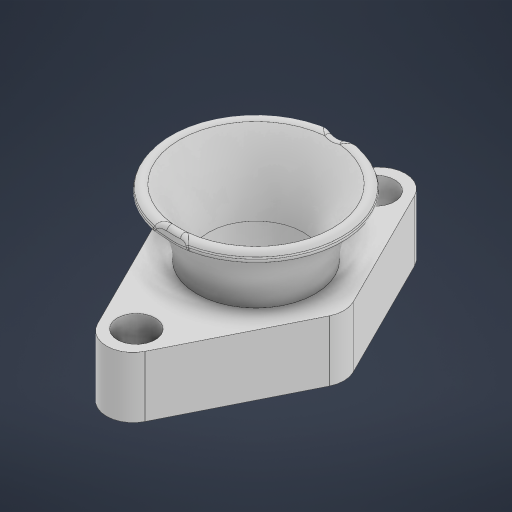
# Autodesk Inventor part: velocity stack
Saved by Autodesk Inventor 2024.2 (Build 282272000, 272)
## iProperties
Created: 2025-06-20
Part Number: velocity stack
Material: Generic
Document SubType Name: Modeling
Designer: Moe
Density: 1 g/cm^3
Appearance: Default
Author: Moe
Autodesk Inventor part; units mm, degrees
ref_plane "YZ Plane" through (0, 0, 0) normal (1, 0, 0) x (0, 1, 0)
ref_plane "XZ Plane" through (0, 0, 0) normal (0, 1, 0) x (-1, 0, 0)
sketch "Sketch1" plane through (0, 0, 0) normal (0, 1, 0) x (-1, 0, 0)
  circle A0 centre (0, 0) radius 6.25
  circle A1 centre (0, -15.75) radius 2.5
  circle A2 centre (0, 15.75) radius 2.5
  line L0 (0, 0) -> (0, -24)
  line L1 (0, 0) -> (0, 24)
  line L2 (0, 0) -> (12, 0)
  line L3 (0, 0) -> (-12, 0)
  line L4 (0, 24) -> (12, 0)
  line L5 (12, 0) -> (0, -24)
  line L6 (0, -24) -> (-12, 0)
  line L7 (-12, 0) -> (0, 24)
  line L8 (12.016091, 26.451229) -> (-11.988013, 26.451229)
  line L9 (-11.988013, 26.451229) -> (-11.988013, 27.744681)
  line L10 (-11.988013, 27.744681) -> (12.016091, 27.744681)
  line L11 (12.016091, 27.744681) -> (12.016091, 26.451229)
  dimension "d0" = 12.5
  dimension "d1" = 5
  dimension "d2" = 5
  dimension "d3" = 15.75
  dimension "d4" = 15.75
  dimension "d5" = 24
  dimension "d6" = 24
  dimension "d7" = 12
  dimension "d8" = 12
  constraints: 24 end point, 3 centre point, 3 horizontal, 2 parallel, 2 vertical, 1 coincident, 1 perpendicular
  measures "d0" diameter of A0
  measures "d1" diameter of A1
  measures "d2" diameter of A2
  measures "d3" distance of point (0, 0) A2.centre
  measures "d4" distance of A1.centre point (0, 0)
  measures "d5" distance of L0.start L0.end
  measures "d6" distance of L0.start L1.end
  measures "d7" distance of L0.start L2.end
  measures "d8" distance of L0.start L3.end
extrude "Extrusion1" add sketch "Sketch1" along normal blind 8 contours L2 L5 L0 A1 A0 | A0 L1 A2 L4 L2 | A0 L3 L7 L1 A2 | L0 A1 L6 L3 A0
fillet "Fillet1" radius 3.5 4 edges at (0, 4, 24) (0, 4, -24) (12, 4, 0) (-12, 4, 0)
sketch "Sketch2" plane through (0, 0, 0) normal (0, -1, 0) x (1, 0, 0)
  circle A0 centre (0, 0) radius 6.25 projected
  circle A1 centre (0, 0) radius 10
  dimension "d12" = 20
  constraints: 1 centre point, 1 coincident
  measures "d12" diameter of A1
extrude "Extrusion2" cut sketch "Sketch2" against normal blind 3.5
extrude "Extrusion3" add sketch "Sketch1" along normal blind 10 contours L8 L9 L10 L11
ref_plane "Work Plane2" through (11.988013, 0, 0.000229) normal (0, 0, -1) x (-1, 0, 0)
extrude "Extrusion4" cut sketch "Sketch1" along normal blind 10 contours L8 L9 L10 L11
sketch "Sketch4" plane through (11.988013, 0, 0.000229) normal (0, 0, -1) x (-1, 0, 0)
  line L0 (23.205389, 8) -> (23.205389, 8)
  line L1 (23.205389, 8) -> (15.118508, 8)
  line L2 (8.857518, 8) -> (15.118508, 8)
  line L3 (8.857518, 8) -> (0.770637, 8)
  line L4 (0.770637, 8) -> (0.770637, 8)
  line L5 (0.770637, 8) -> (8.857518, 8)
  line L6 (15.118508, 8) -> (8.857518, 8)
  line L7 (15.118508, 8) -> (23.205389, 8)
  line L8 (9.488013, 8) -> (14.488013, 8)
  line L9 (9.488013, 8) -> (14.488013, 8)
  line L10 (5.738013, 8) -> (18.238013, 8)
  line L11 (5.738013, 3.5) -> (18.238013, 3.5)
  line L12 (5.738013, 8) -> (18.238013, 8)
  arc A0 (22.062221, 16.642429) -> (18.238013, 8) centre (29.105693, 8.358441) ccw
  line L13 (18.238013, 8) -> (23.982272, 17.949349) construction
  line L14 (18.238013, 8) -> (29.726531, 8) construction
  line L15 (23.205389, 8) -> (15.118508, 8)
  line L16 (19.793316, 8) -> (18.238013, 8)
  line L17 (11.988013, 0) -> (11.988013, 10.466692)
  arc A1 (23.281166, 15.663138) -> (19.779795, 7.800469) centre (29.105693, 8.358441) ccw
  line L18 (23.326048, 16.322868) -> (23.4046, 16.120844)
  arc A2 (23.326048, 16.322868) -> (22.062221, 16.642429) centre (22.580428, 16.032953) ccw
  arc A3 (23.281166, 15.663138) -> (23.4046, 16.120844) centre (23.03179, 15.975886) ccw
  point P0 (22.940237, 17.31512)
  point P1 (23.512979, 15.842108)
  point P2 (19.769997, 8)
  dimension "d22" = 60
  dimension "d26" = 0.8
  dimension "d27" = 0.4
  constraints: 11 point on circle, 10 end point, 4 centre point, 4 tangent, 3 point on line, 1 coincident, 1 collinear, 1 equal length, 1 horizontal, 1 vertical
  measures "d22" angle of L14 L13
  measures "d26" radius of A2
  measures "d27" radius of A3
revolve "Revolution1" add sketch "Sketch4" angle 360 about axis through (0, 0, 0.000229) along (0, 1, 0)
sketch "Sketch5" plane through (0, 8, 0) normal (0, 1, 0) x (1, 0, 0)
  circle A0 centre (0, -15.75) radius 2.5
  circle A1 centre (0, 15.75) radius 2.5
  arc A2 (-11.217376, 1.565248) -> (-11.217376, -1.565248) centre (-8.086881, 0) ccw
  line L0 (-11.217376, -1.565248) -> (-3.130495, -17.73901)
  arc A3 (-3.130495, -17.73901) -> (3.130495, -17.73901) centre (0, -16.173762) ccw
  line L1 (3.130495, -17.73901) -> (11.217376, -1.565248)
  arc A4 (11.217376, -1.565248) -> (11.217376, 1.565248) centre (8.086881, 0) ccw
  line L2 (11.217376, 1.565248) -> (3.130495, 17.73901)
  arc A5 (3.130495, 17.73901) -> (-3.130495, 17.73901) centre (0, 16.173762) ccw
  line L3 (-3.130495, 17.73901) -> (-11.217376, 1.565248)
  circle A6 centre (0, -0.000229) radius 7.781984
  circle A7 centre (0, 15.75) radius 5
  circle A8 centre (0, -15.75) radius 5
  point P0 (0, 0)
  dimension "d28" = 10
  dimension "d29" = 10
  constraints: 2 centre point, 2 coincident
  measures "d28" diameter of A7
  measures "d29" diameter of A8
extrude "Extrusion5" cut sketch "Sketch5" along normal blind 10 contours A0 | A1 | A7 L2 A5 L3 | L3 A5 L2 A7 | A8 L1 A3 L0 | L0 A3 L1 A8
fillet "Fillet3" radius 0.5 12 edges at (-2.0519, 16.222, -11.1904) (-2.1336, 15.8689, -11.2281) (0, 15.1951, -10.75) (2.1336, 15.8689, -11.2281) (2.0519, 16.222, -11.1904) (0, 16.8172, -10.75) (2.0527, 16.222, 11.1908) (2.1343, 15.8689, 11.2284) (0, 15.1946, 10.75) (-2.1343, 15.8689, 11.2284) (-2.0527, 16.222, 11.1908) (0, 16.8173, 10.75)
body "Solid1"
